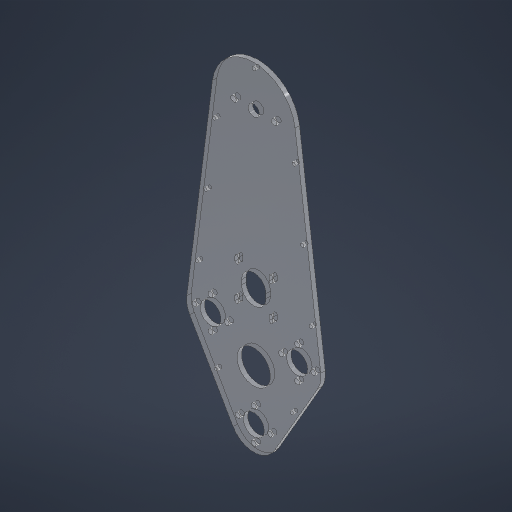
# Autodesk Inventor part: 1ELO
Saved by Autodesk Inventor 2025.2 (Build 292293000, 293)
## iProperties
Created: 2025-05-02
Part Number: 1ELO
Material: Generic
Document SubType Name: Modeling
Designer: Nelson
Density: 1 g/cm^3
Appearance: Polycarbonate - Clear
Author: Nelson
Autodesk Inventor part; units mm, degrees
ref_plane "YZ Plane" through (0, 0, 0) normal (1, 0, 0) x (0, 1, 0)
ref_plane "XZ Plane" through (0, 0, 0) normal (0, 1, 0) x (-1, 0, 0)
ref_plane "XY Plane" through (0, 0, 0) normal (0, 0, 1) x (1, 0, 0)
sketch "Sketch1" plane through (0, 0, 0) normal (0, 0, 1) x (1, 0, 0)
  line L0 (0, 0) -> (0, 200) construction
  arc A0 (37.1934, 204.7857) -> (-37.1934, 204.7857) centre (0, 200) ccw
  line L1 (0, 200) -> (-18.25, 200) construction
  circle A1 centre (-18.25, 200) radius 2.5
  line L2 (0, 200) -> (18.25, 200) construction
  circle A2 centre (18.25, 200) radius 2.5
  circle A3 centre (0, 0) radius 15
  line L3 (37.1934, 204.7857) -> (59.7122, 29.7756)
  line L4 (-37.1934, 204.7857) -> (-59.9286, 28.0941)
  line L5 (48.4528, 117.2807) -> (43.4937, 116.6426) construction
  line L6 (51.1509, 57.1332) -> (35.8365, 176.152) construction
  circle A4 centre (35.8365, 176.152) radius 1.5
  circle A5 centre (51.1509, 57.1332) radius 1.5
  circle A6 centre (43.4937, 116.6426) radius 1.5
  line L7 (0, 237.5) -> (0, 232.5) construction
  circle A7 centre (0, 232.5) radius 1.5
  circle A8 centre (-35.8365, 176.152) radius 1.5
  circle A9 centre (-51.1509, 57.1332) radius 1.5
  circle A10 centre (-43.4937, 116.6426) radius 1.5
  circle A11 centre (0, 200) radius 5
  line L8 (0, 200) -> (0, 60.58) construction
  circle A12 centre (0, 60.58) radius 11 construction
  line L9 (0, 62.58) -> (0, 58.58) construction
  arc A13 (-11, 58.58) -> (11, 58.58) centre (0, 58.58) ccw
  line L10 (-11, 62.58) -> (-11, 58.58)
  line L11 (11, 62.58) -> (11, 58.58)
  arc A14 (11, 62.58) -> (-11, 62.58) centre (0, 62.58) ccw
  line L12 (-15.5, 60.58) -> (15.5, 60.58) construction
  line L13 (0, 76.08) -> (0, 45.08) construction
  circle A15 centre (-15.5, 45.08) radius 1.5 construction
  line L14 (-15.5, 47.08) -> (-15.5, 43.08) construction
  arc A16 (-14, 47.08) -> (-16.9989, 47.0217) centre (-15.5, 47.08) ccw
  line L15 (-14, 47.08) -> (-14, 43.08)
  line L16 (-17, 43.08) -> (-17, 47.08)
  arc A17 (-17, 43.08) -> (-14, 43.08) centre (-15.5, 43.08) ccw
  circle A18 centre (15.5, 45.08) radius 1.5 construction
  line L17 (15.5, 47.08) -> (15.5, 43.08) construction
  arc A19 (16.9989, 47.0217) -> (14, 47.08) centre (15.5, 47.08) ccw
  line L18 (14, 47.08) -> (14, 43.08)
  line L19 (17, 43.08) -> (17, 47.08)
  arc A20 (14, 43.08) -> (17, 43.08) centre (15.5, 43.08) ccw
  circle A21 centre (-15.5, 76.08) radius 1.5 construction
  line L20 (-15.5, 74.08) -> (-15.5, 78.08) construction
  arc A22 (-16.9989, 74.1383) -> (-14, 74.08) centre (-15.5, 74.08) ccw
  line L21 (-14, 74.08) -> (-14, 78.08)
  line L22 (-17, 78.08) -> (-17, 74.08)
  arc A23 (-14, 78.08) -> (-17, 78.08) centre (-15.5, 78.08) ccw
  arc A24 (17, 78.08) -> (14, 78.08) centre (15.5, 78.08) ccw
  circle A25 centre (15.5, 76.08) radius 1.5 construction
  line L23 (14, 74.08) -> (14, 78.08)
  line L24 (15.5, 74.08) -> (15.5, 78.08) construction
  line L25 (17, 78.08) -> (17, 74.08)
  arc A26 (14, 74.08) -> (16.9989, 74.1383) centre (15.5, 74.08) ccw
  circle A27 centre (0, 0) radius 45 construction
  circle A28 centre (0, -45) radius 9.5
  circle A29 centre (0, -45) radius 14.5 construction
  circle A30 centre (0, -59.5) radius 2.25
  circle A31 centre (14.5, -45) radius 2.25
  circle A32 centre (0, -30.5) radius 2.25
  circle A33 centre (-14.5, -45) radius 2.25
  circle A34 centre (0, -45) radius 21.5 construction
  circle A35 centre (38.9711, 22.5) radius 21.5 construction
  circle A36 centre (51.5285, 29.75) radius 2.25 construction
  circle A37 centre (46.2211, 9.9426) radius 2.25 construction
  circle A38 centre (31.7211, 35.0574) radius 2.25 construction
  circle A39 centre (26.4138, 15.25) radius 2.25 construction
  circle A40 centre (38.9711, 22.5) radius 9.5
  circle A41 centre (-38.9711, 22.5) radius 21.5 construction
  circle A42 centre (-51.5285, 29.75) radius 2.25 construction
  circle A43 centre (-31.7211, 35.0574) radius 2.25 construction
  circle A44 centre (-46.2211, 9.9426) radius 2.25 construction
  circle A45 centre (-26.4138, 15.25) radius 2.25 construction
  circle A46 centre (-38.9711, 22.5) radius 9.5
  line L26 (-18.6195, -55.75) -> (-57.5907, 11.75)
  line L27 (18.6195, -55.75) -> (57.5907, 11.75)
  line L28 (48.4528, 117.2807) -> (48.4528, 23.0901) construction
  line L29 (59.7122, 29.7756) -> (60.2953, 25.2438)
  line L30 (48.4528, 23.0901) -> (48.4528, -26.9099) construction
  line L31 (48.4528, -26.9099) -> (38.566, -21.2018) construction
  line L32 (38.566, -21.2018) -> (34.2359, -18.7018) construction
  circle A47 centre (34.2359, -18.7018) radius 1.5
  circle A48 centre (-34.2359, -18.7018) radius 1.5
  arc A49 (57.5907, 11.75) -> (60.2953, 25.2438) centre (38.9711, 22.5) ccw
  arc A50 (-60.2953, 25.2438) -> (-57.5907, 11.75) centre (-38.9711, 22.5) ccw
  arc A51 (-18.6195, -55.75) -> (18.6195, -55.75) centre (0, -45) ccw
  circle A52 centre (38.9711, 22.5) radius 14.5 construction
  circle A53 centre (53.4711, 22.5) radius 2.25
  line L33 (38.9711, 22.5) -> (53.4711, 22.5) construction
  circle A54 centre (38.9711, 37) radius 2.25
  circle A55 centre (24.4711, 22.5) radius 2.25
  circle A56 centre (38.9711, 8) radius 2.25
  circle A57 centre (-53.4711, 22.5) radius 2.25
  circle A58 centre (-38.9711, 37) radius 2.25
  circle A59 centre (-24.4711, 22.5) radius 2.25
  circle A60 centre (-38.9711, 8) radius 2.25
  line L34 (-59.9286, 28.0941) -> (-60.2953, 25.2438)
  dimension "d79" = 90
  dimension "d81" = 29
  dimension "d99" = 29
  dimension "L_Elo" = 200
  dimension "D_Junta2" = 75
  dimension "d13" = 18.25
  dimension "d14" = 5
  dimension "D_furoZ" = 30
  dimension "d16" = 5
  dimension "d17" = 120
  dimension "d18" = 3
  dimension "d19" = 3
  dimension "d20" = 3
  dimension "d21" = 5
  dimension "d22" = 3
  dimension "D_Eixo" = 10
  dimension "CA" = 139.42
  dimension "DN" = 22
  dimension "NN" = 4
  dimension "d51" = 22
  dimension "d53" = 11
  dimension "d54" = 31
  dimension "d55" = 31
  dimension "FN" = 3
  dimension "d57" = 15.5
  dimension "d58" = 15.5
  dimension "d59" = 4
  dimension "d61" = 3
  dimension "d62" = 1.5
  dimension "d80" = 19
  dimension "d82" = 4.5
  dimension "d83" = 45
  dimension "d84" = 14.5
  dimension "d85" = 14.5
  dimension "d88" = 360
  dimension "d90" = 43
  dimension "d93" = 360
  dimension "d95" = 94.1906
  dimension "d96" = 50
  dimension "d97" = 5
  dimension "d98" = 3
  dimension "d100" = 4.5
  dimension "d104" = 360
  constraints: 70 end point, 57 centre point, 40 symmetric about line, 39 point on circle, 26 coincident, 20 tangent, 6 midpoint, 6 point on line, 6 vertical alignment, 4 vertical, 3 horizontal, 3 horizontal alignment, 2 concentric, 2 perpendicular, 1 collinear, 1 parallel, 82 other
  measures "L_Elo" distance of L0.start L0.end
  measures "D_Junta2" diameter of A0
  measures "d13" distance of L1.start L1.end
  measures "d14" diameter of A1
  measures "D_furoZ" diameter of A3
  measures "d16" distance of L5.start L5.end
  measures "d17" distance of L6.start L6.end
  measures "d18" diameter of A4
  measures "d19" diameter of A5
  measures "d20" diameter of A6
  measures "d21" distance of L7.start L7.end
  measures "d22" diameter of A7
  measures "D_Eixo" diameter of A11
  measures "CA" distance of L8.start L8.end
  measures "DN" diameter of A12
  measures "NN" distance of L9.start L9.end
  measures "d51" diameter of A13
  measures "d53" radius of A14
  measures "d54" distance of L12.start L12.end
  measures "d55" distance of L13.start L13.end
  measures "FN" diameter of A15
  measures "d57" distance of A15.centre L13.end
  measures "d58" distance of L12.start A15.centre
  measures "d59" distance of L14.start L14.end
  measures "d61" diameter of A16
  measures "d62" radius of A17
  measures "d80" diameter of A28
  measures "d82" diameter of A30
  measures "d83" distance of point (0, 0) A28.centre
  measures "d84" distance of A28.centre A30.centre
  measures "d85" distance of A30.centre point (0, -45)
  measures "d90" diameter of A34
  measures "d95" distance of L5.start L28.end
  measures "d96" distance of L28.end L30.end
  measures "d97" distance of L31.end L32.end
  measures "d98" diameter of A47
  measures "d100" diameter of A53
extrude "Extrusion1" add sketch "Sketch1" along normal blind 4
equation "\"d16\" = LF"
equation "\"d18\" = D_Sup"
equation "\"d19\" = D_Sup"
equation "\"d20\" = D_Sup"
equation "\"d21\" = LF"
equation "\"d22\" = D_Sup"
equation "\"LF\" = 5"
equation "\"D_Sup\" = 3"
body "Solid1"
